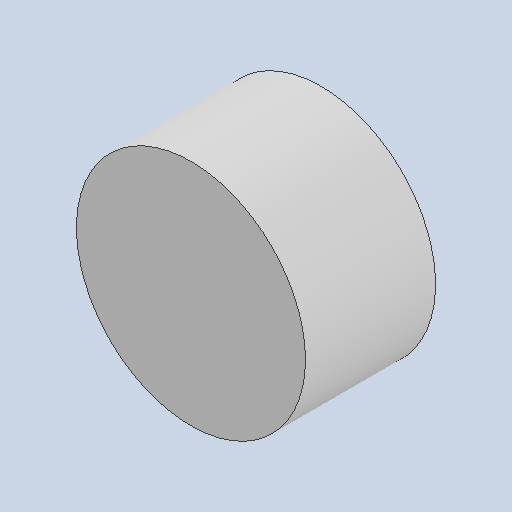
# Autodesk Inventor part: opona
Saved by Autodesk Inventor 2023 (Build 270158000, 158)
## iProperties
Created: 2022-12-13
Part Number: opona
Material: Generic
Document SubType Name: Modeling
Designer: komputer
Density: 1 g/cm^3
Appearance: Default
Author: komputer
Autodesk Inventor part; units mm, degrees
ref_plane "YZ Plane" through (0, 0, 0) normal (1, 0, 0) x (0, 1, 0)
sketch "Sketch1" plane through (0, 0, 0) normal (0, 0, 1) x (1, 0, 0)
  circle A0 centre (-10, 3.96) radius 8 projected
  line L0 (-10, 3.96) -> (-10, -7.04)
  circle A1 centre (-10, 3.96) radius 11
  point P0 (0, 0)
  dimension "d0" = 11
  constraints: 2 end point, 1 coincident, 1 vertical, 1 vertical alignment, 2 other
  measures "d0" distance of L0.start L0.end
ref_plane "Work Plane1" through (-18, -4.04, -12.5) normal (0, 0, -1) x (0, 1, 0)
extrude "Extrusion1" add sketch "Sketch1" against normal up to surface (12.5 mm away)
sketch "Sketch2" plane through (-10, 3.96, 0) normal (0, 0, 1) x (1, 0, 0)
  circle A0 centre (0, 0) radius 11 projected
  circle A1 centre (0, 0) radius 8 projected
  point P0 (10, -3.96)
ref_plane "Work Plane2" through (-18, -4.04, -3.5) normal (0, 0, 1) x (1, 0, 0)
extrude "Extrusion2" add sketch "Sketch2" against normal up to surface (3.5 mm away) contours A1
body "Solid1"
